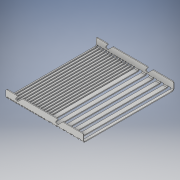
# Autodesk Inventor part: Einschub
Saved by Autodesk Inventor 2018 (Build 220112000, 112)
## iProperties
Created: 2017-12-09
Part Number: Einschub
Material: Generisch
Document SubType Name: Blech
Designer: aXe
Density: 1 g/cm^3
Sheet Metal Rule: Standard_mm
Appearance: Vorgabe
Flat Pattern Width: 19.3 cm
Flat Pattern Length: 26.0048 cm
Flat Pattern Area: 501.892 cm^2
Sheet Metal Width: 193,000 mm
Sheet Metal Length: 260,048 mm
Sheet Metal Area: 50189,223 mm^2
Author: aXe
Autodesk Inventor part; units mm, degrees
ref_plane "YZ Plane" through (0, 0, 0) normal (1, 0, 0) x (0, 1, 0)
ref_plane "XZ Plane" through (0, 0, 0) normal (0, 1, 0) x (-1, 0, 0)
ref_plane "XY Plane" through (0, 0, 0) normal (0, 0, 1) x (1, 0, 0)
sketch "Skizze1 outline for Grobblech1" plane through (0, 0, 0) normal (0, 0, 1) x (1, 0, 0)
  line L0 (154, 22) -> (154, 245)
  line L1 (-39, 22) -> (154, 22)
  line L2 (-39, 245) -> (-39, 22)
  line L3 (154, 245) -> (-39, 245)
extrude "Grobblech1" add sketch "Skizze1 outline for Grobblech1" along normal blind 2
sketch "Skizze3" plane through (-39, 245, 2) normal (0, 1, 0) x (-1, 0, 0)
  line L0 (-193, 0) -> (0, 0)
  line L1 (0, 0) -> (0, 18)
  line L2 (0, 18) -> (-193, 18)
  line L3 (-193, 18) -> (-193, 0)
  constraints: 6 end point, 1 horizontal, 1 perpendicular, 1 vertical
edge flange "Lasche2" height 20 angle 90 thickness 2 bend radius 2 thickness toward (0, 1, 0) relief tear relief width 2 relief depth 1 corner gap 2 corner form 0 edges at (57.5, 245, 2) (57.5, 22, 2) wall of the first edge with corners at (154, 245, 2) (-39, 245, 2) (-39, 245, 20) (154, 245, 20)
bend "Biegung2"
corner "Ecke2"
sketch "Skizze1" plane through (0, 0, 0) normal (0, 0, 1) x (1, 0, 0)
  line L0 (-54, 29.504008) -> (-54, 245.504008)
  line L1 (-14.2, 22) -> (-7.8, 22)
  line L2 (-7.8, 245) -> (-14.2, 245)
  line L3 (92.2, 245) -> (85.8, 245)
  line L4 (85.8, 22) -> (92.2, 22)
  line L5 (204, 8.1) -> (204, 258.9)
  line L6 (154, 245) -> (-39, 245)
  line L7 (-39, 245) -> (-39, 22)
  line L8 (-39, 22) -> (154, 22)
  line L9 (154, 22) -> (154, 245)
  point P0 (0, 0)
  dimension "d0" = 0
  dimension "d1" = 0
  dimension "d2" = 15
  dimension "d3" = 50
  measures "d0" distance between parallel lines of L1 L8
  measures "d1" distance between parallel lines of L2 L6
  measures "d2" distance between parallel lines of L0 L7
  measures "d3" distance between parallel lines of L5 L9
sketch "Skizze4" plane through (-39, 247, 20) normal (0, 1, 0) x (1, 0, 0)
  circle A0 centre (28, 8.499917) radius 3.5 construction
  circle A1 centre (28, 8.499917) radius 3.65 construction
  line L0 (28, 8.499917) -> (42.660327, -6.16041) construction
  line L1 (25.41906, 5.918977) -> (40.079388, -8.74135)
  line L2 (45.241267, -3.579471) -> (30.58094, 11.080857)
  arc A2 (30.58094, 11.080857) -> (25.41906, 5.918977) centre (28, 8.499917) ccw
  arc A3 (40.079388, -8.74135) -> (45.241267, -3.579471) centre (42.660327, -6.16041) ccw
  line L3 (28, 8.499917) -> (48.732834, 8.499917) construction
  circle A4 centre (128, 8.499917) radius 3.5 construction
  circle A5 centre (128, 8.499917) radius 3.65 construction
  line L4 (128, 8.499917) -> (142.660327, -6.16041) construction
  line L5 (125.41906, 5.918977) -> (140.079388, -8.74135)
  line L6 (145.241267, -3.579471) -> (130.58094, 11.080857)
  arc A6 (130.58094, 11.080857) -> (125.41906, 5.918977) centre (128, 8.499917) ccw
  arc A7 (140.079388, -8.74135) -> (145.241267, -3.579471) centre (142.660327, -6.16041) ccw
  line L7 (128, 8.499917) -> (148.732834, 8.499917) construction
  point P0 (39, 20)
  point P1 (35.330164, 1.169753)
  point P2 (135.330164, 1.169753)
  dimension "d25" = 0.15
  dimension "d26" = 45
  dimension "d27" = 45
  dimension "d28" = 59.70035
  constraints: 20 end point, 8 point on circle, 8 tangent, 6 centre point, 3 equal radius, 3 parallel, 2 equal length, 2 horizontal, 2 midpoint, 1 concentric
  measures "d25" radial gap between concentric circles of A0 A1
  measures "d26" angle of L0 L3
  measures "d27" angle of L4 L7
  measures "d28" distance from line of L3.end L6
sketch "Skizze4 outline for Extrusion1" plane through (-39, 247, 20) normal (0, 1, 0) x (1, 0, 0)
  arc A0 (30.58094, 11.080857) -> (25.41906, 5.918977) centre (28, 8.499917) ccw
  line L0 (45.241267, -3.579471) -> (30.58094, 11.080857)
  arc A1 (40.079388, -8.74135) -> (45.241267, -3.579471) centre (42.660327, -6.16041) ccw
  line L1 (25.41906, 5.918977) -> (40.079388, -8.74135)
  arc A2 (130.58094, 11.080857) -> (125.41906, 5.918977) centre (128, 8.499917) ccw
  line L2 (145.241267, -3.579471) -> (130.58094, 11.080857)
  arc A3 (140.079388, -8.74135) -> (145.241267, -3.579471) centre (142.660327, -6.16041) ccw
  line L3 (125.41906, 5.918977) -> (140.079388, -8.74135)
extrude "Extrusion1" cut sketch "Skizze4 outline for Extrusion1" against normal through all
fillet "Rundung1" radius 2 4 edges at (-7.662, 246, 20) (2.6618, 246, 20) (92.338, 246, 20) (102.6618, 246, 20)
fillet "Rundung2" radius 2 4 edges at (2.6618, 21, 20) (-7.662, 21, 20) (92.338, 21, 20) (102.6618, 21, 20)
sketch "Skizze5" plane through (-39, 20, 4) normal (0, -1, 0) x (1, 0, 0)
  line L0 (-175.560035, -4) -> (344.260006, -4)
  line L1 (0, 0) -> (0, -4) construction
  line L2 (0, 0) -> (0, 16) construction
  line L3 (193, -4) -> (193, 0) construction
  line L4 (193, 16) -> (193, 0) construction
  line L5 (3, -4) -> (6, -4)
  line L6 (6, -4) -> (6, 1)
  line L7 (6, 1) -> (3, 1)
  line L8 (3, 1) -> (3, -4)
  line L9 (10, -4) -> (13, -4)
  line L10 (13, -4) -> (13, 1)
  line L11 (13, 1) -> (10, 1)
  line L12 (10, 1) -> (10, -4)
  line L13 (17, -4) -> (20, -4)
  line L14 (20, -4) -> (20, 1)
  line L15 (20, 1) -> (17, 1)
  line L16 (17, 1) -> (17, -4)
  line L17 (24, -4) -> (27, -4)
  line L18 (27, -4) -> (27, 1)
  line L19 (27, 1) -> (24, 1)
  line L20 (24, 1) -> (24, -4)
  line L21 (31, -4) -> (34, -4)
  line L22 (34, -4) -> (34, 1)
  line L23 (34, 1) -> (31, 1)
  line L24 (31, 1) -> (31, -4)
  line L25 (38, -4) -> (41, -4)
  line L26 (41, -4) -> (41, 1)
  line L27 (41, 1) -> (38, 1)
  line L28 (38, 1) -> (38, -4)
  line L29 (45, -4) -> (48, -4)
  line L30 (48, -4) -> (48, 1)
  line L31 (48, 1) -> (45, 1)
  line L32 (45, 1) -> (45, -4)
  line L33 (52, -4) -> (55, -4)
  line L34 (55, -4) -> (55, 1)
  line L35 (55, 1) -> (52, 1)
  line L36 (52, 1) -> (52, -4)
  line L37 (59, -4) -> (62, -4)
  line L38 (62, -4) -> (62, 1)
  line L39 (62, 1) -> (59, 1)
  line L40 (59, 1) -> (59, -4)
  line L41 (66, -4) -> (69, -4)
  line L42 (69, -4) -> (69, 1)
  line L43 (69, 1) -> (66, 1)
  line L44 (66, 1) -> (66, -4)
  line L45 (73, 1) -> (73, -4)
  line L46 (73, -4) -> (76, -4)
  line L47 (76, -4) -> (76, 1)
  line L48 (76, 1) -> (73, 1)
  line L49 (80, 1) -> (80, -4)
  line L50 (80, -4) -> (83, -4)
  line L51 (83, -4) -> (83, 1)
  line L52 (83, 1) -> (80, 1)
  line L53 (87, 1) -> (87, -4)
  line L54 (87, -4) -> (90, -4)
  line L55 (90, -4) -> (90, 1)
  line L56 (90, 1) -> (87, 1)
  line L57 (94, 1) -> (94, -4)
  line L58 (94, -4) -> (97, -4)
  line L59 (97, -4) -> (97, 1)
  line L60 (97, 1) -> (94, 1)
  line L61 (107, -4) -> (115, -4)
  line L62 (115, -4) -> (115, 1)
  line L63 (115, 1) -> (107, 1)
  line L64 (107, 1) -> (107, -4)
  line L65 (133, -4) -> (133, 1)
  line L66 (125, -4) -> (133, -4)
  line L67 (125, 1) -> (125, -4)
  line L68 (133, 1) -> (125, 1)
  line L69 (151, -4) -> (151, 1)
  line L70 (143, -4) -> (151, -4)
  line L71 (143, 1) -> (143, -4)
  line L72 (151, 1) -> (143, 1)
  line L73 (169, -4) -> (169, 1)
  line L74 (161, -4) -> (169, -4)
  line L75 (161, 1) -> (161, -4)
  line L76 (169, 1) -> (161, 1)
  line L77 (187, -4) -> (187, 1)
  line L78 (179, -4) -> (187, -4)
  line L79 (179, 1) -> (179, -4)
  line L80 (187, 1) -> (179, 1)
  point P0 (39, -4)
  dimension "d33" = 5
  dimension "d34" = 3
  dimension "d35" = 0
  dimension "d36" = 3
  dimension "d39" = 7
  dimension "d46" = 7
  dimension "d51" = 5
  dimension "d52" = 8
  dimension "d53" = 0
  dimension "d54" = 10
  dimension "d57" = 18
  constraints: 154 end point, 6 horizontal, 4 parallel, 2 perpendicular, 138 other
  measures "d33" distance between parallel lines of L7 L5
  measures "d34" distance between parallel lines of L8 L6
  measures "d35" distance between parallel lines of L0 L5
  measures "d36" distance between parallel lines of L1 L8
  measures "d39" distance of L5.start L9.start
  measures "d46" distance of L41.start L45.end
  measures "d51" distance between parallel lines of L63 L61
  measures "d52" distance between parallel lines of L64 L62
  measures "d53" distance between parallel lines of L0 L61
  measures "d54" distance between parallel lines of L59 L64
  measures "d57" distance of L62.end L65.end
sketch "Skizze5 outline for Extrusion2" plane through (-39, 20, 4) normal (0, -1, 0) x (1, 0, 0)
  line L0 (3, 1) -> (3, -4)
  line L1 (6, 1) -> (3, 1)
  line L2 (6, -4) -> (6, 1)
  line L3 (3, -4) -> (6, -4)
  line L4 (10, 1) -> (10, -4)
  line L5 (13, 1) -> (10, 1)
  line L6 (13, -4) -> (13, 1)
  line L7 (10, -4) -> (13, -4)
  line L8 (17, 1) -> (17, -4)
  line L9 (20, 1) -> (17, 1)
  line L10 (20, -4) -> (20, 1)
  line L11 (17, -4) -> (20, -4)
  line L12 (24, 1) -> (24, -4)
  line L13 (27, 1) -> (24, 1)
  line L14 (27, -4) -> (27, 1)
  line L15 (24, -4) -> (27, -4)
  line L16 (31, 1) -> (31, -4)
  line L17 (34, 1) -> (31, 1)
  line L18 (34, -4) -> (34, 1)
  line L19 (31, -4) -> (34, -4)
  line L20 (38, 1) -> (38, -4)
  line L21 (41, 1) -> (38, 1)
  line L22 (41, -4) -> (41, 1)
  line L23 (38, -4) -> (41, -4)
  line L24 (45, 1) -> (45, -4)
  line L25 (48, 1) -> (45, 1)
  line L26 (48, -4) -> (48, 1)
  line L27 (45, -4) -> (48, -4)
  line L28 (52, 1) -> (52, -4)
  line L29 (55, 1) -> (52, 1)
  line L30 (55, -4) -> (55, 1)
  line L31 (52, -4) -> (55, -4)
  line L32 (59, 1) -> (59, -4)
  line L33 (62, 1) -> (59, 1)
  line L34 (62, -4) -> (62, 1)
  line L35 (59, -4) -> (62, -4)
  line L36 (66, 1) -> (66, -4)
  line L37 (69, 1) -> (66, 1)
  line L38 (69, -4) -> (69, 1)
  line L39 (66, -4) -> (69, -4)
  line L40 (73, 1) -> (73, -4)
  line L41 (76, 1) -> (73, 1)
  line L42 (76, -4) -> (76, 1)
  line L43 (73, -4) -> (76, -4)
  line L44 (80, 1) -> (80, -4)
  line L45 (83, 1) -> (80, 1)
  line L46 (83, -4) -> (83, 1)
  line L47 (80, -4) -> (83, -4)
  line L48 (87, 1) -> (87, -4)
  line L49 (90, 1) -> (87, 1)
  line L50 (90, -4) -> (90, 1)
  line L51 (87, -4) -> (90, -4)
  line L52 (94, 1) -> (94, -4)
  line L53 (97, 1) -> (94, 1)
  line L54 (97, -4) -> (97, 1)
  line L55 (94, -4) -> (97, -4)
  line L56 (107, 1) -> (107, -4)
  line L57 (115, 1) -> (107, 1)
  line L58 (115, -4) -> (115, 1)
  line L59 (107, -4) -> (115, -4)
  line L60 (133, 1) -> (133, -4)
  line L61 (133, -4) -> (125, -4)
  line L62 (125, -4) -> (125, 1)
  line L63 (125, 1) -> (133, 1)
  line L64 (151, 1) -> (151, -4)
  line L65 (151, -4) -> (143, -4)
  line L66 (143, -4) -> (143, 1)
  line L67 (143, 1) -> (151, 1)
  line L68 (169, 1) -> (169, -4)
  line L69 (169, -4) -> (161, -4)
  line L70 (161, -4) -> (161, 1)
  line L71 (161, 1) -> (169, 1)
  line L72 (187, 1) -> (187, -4)
  line L73 (187, -4) -> (179, -4)
  line L74 (179, -4) -> (179, 1)
  line L75 (179, 1) -> (187, 1)
extrude "Extrusion2" cut sketch "Skizze5 outline for Extrusion2" against normal through all
fillet "Rundung3" radius 2 4 edges at (154, 21, 20) (-39, 21, 20) (-39, 246, 20) (154, 246, 20)
equation "\"d4\" = Stärke"
equation "\"d15\" = BreiteBiegungsfreistellung"
equation "\"d16\" = TiefeBiegungsfreistellung"
equation "\"d17\" = MinimalRest"
equation "\"d18\" = Übergangsradius"
equation "\"d21\" = Biegeradius"
equation "\"d22\" = GrößeEckenfreistellung"
equation "\"d23\" = Abstandsgröße"
equation "\"d24\" = JacobiRadiusGröße"
equation "\"Biegeradius\" = Stärke"
equation "\"BreiteBiegungsfreistellung\" = Stärke"
equation "\"TiefeBiegungsfreistellung\" = 0.5 * Stärke"
equation "\"GrößeEckenfreistellung\" = 4 * Stärke"
equation "\"MinimalRest\" = 2 * Stärke"
equation "\"Übergangsradius\" = Biegeradius"
equation "\"JacobiRadiusGröße\" = Biegeradius"
equation "\"Abstandsgröße\" = Stärke"
equation "\"Stärke\" = 2"
